Autodesk Fusion 360 part; units mm, degrees
(part 4 of 4)
sketch "Esboço11" plane through (0, 0, 2) normal (0, 0, 1) x (-1, 0, 0)
  circle A0 centre (10.25, -46.6) radius 1.5
  line L0 (8, -42.5) -> (8, -50.7)
  line L1 (8, -50.7) -> (-8, -50.7)
  line L2 (-8, -50.7) -> (-8, -42.5)
  line L3 (-8, -42.5) -> (8, -42.5)
  circle A1 centre (-10.25, -46.6) radius 1.5
  circle A2 centre (40.65, 50) radius 2.15
  arc A3 (-57.5607, 76.943) -> (-64.8173, 70.6939) centre (-60.2496, 72.7276) ccw
  line L4 (-57.5607, 76.943) -> (-49.4611, 71.7764)
  arc A4 (-47.15, 67.561) -> (-49.4611, 71.7764) centre (-52.15, 67.561) ccw
  line L5 (-47.15, 67.561) -> (-47.15, 42.4858)
  arc A5 (-47.4521, 41.7697) -> (-47.15, 42.4858) centre (-48.15, 42.4858) ccw
  line L6 (-47.4521, 41.7697) -> (-49.5538, 39.7214)
  arc A6 (-51.1653, 40.0309) -> (-49.5538, 39.7214) centre (-50.2517, 40.4376) ccw
  line L7 (-51.1653, 40.0309) -> (-64.8173, 70.6939)
  circle A7 centre (-40.65, 50) radius 2.15
  circle A8 centre (40.65, 60) radius 2.15
  line L8 (47.15, 42.4858) -> (47.15, 67.561)
  arc A9 (49.4611, 71.7764) -> (47.15, 67.561) centre (52.15, 67.561) ccw
  line L9 (49.4611, 71.7764) -> (57.5607, 76.943)
  arc A10 (64.8173, 70.6939) -> (57.5607, 76.943) centre (60.2496, 72.7276) ccw
  line L10 (64.8173, 70.6939) -> (51.1653, 40.0309)
  arc A11 (49.5538, 39.7214) -> (51.1653, 40.0309) centre (50.2517, 40.4376) ccw
  line L11 (49.5538, 39.7214) -> (47.4521, 41.7697)
  arc A12 (47.15, 42.4858) -> (47.4521, 41.7697) centre (48.15, 42.4858) ccw
  circle A13 centre (-40.65, 60) radius 2.15
  line L12 (-6.3787, 9) -> (6.3787, 9)
  arc A14 (6.7322, 8.1464) -> (6.3787, 9) centre (6.3787, 8.5) ccw
  line L13 (6.7322, 8.1464) -> (0.7071, 2.1213)
  arc A15 (-0.7071, 2.1213) -> (0.7071, 2.1213) centre (0, 2.8284) ccw
  line L14 (-0.7071, 2.1213) -> (-6.7322, 8.1464)
  arc A16 (-6.3787, 9) -> (-6.7322, 8.1464) centre (-6.3787, 8.5) ccw
  line L15 (-9, -6.3787) -> (-9, 6.3787)
  arc A17 (-8.1464, 6.7322) -> (-9, 6.3787) centre (-8.5, 6.3787) ccw
  line L16 (-8.1464, 6.7322) -> (-2.1213, 0.7071)
  arc A18 (-2.1213, -0.7071) -> (-2.1213, 0.7071) centre (-2.8284, 0) ccw
  line L17 (-2.1213, -0.7071) -> (-8.1464, -6.7322)
  arc A19 (-9, -6.3787) -> (-8.1464, -6.7322) centre (-8.5, -6.3787) ccw
  circle A20 centre (0, 87.5) radius 2.15
  line L18 (-16.4256, 75.2214) -> (0, 81.5)
  line L19 (0, 81.5) -> (15.6612, 75.3836)
  line L20 (41.7895, -17.0192) -> (61.9965, -63.6935)
  arc A21 (55.3948, -68.0303) -> (61.9965, -63.6935) centre (58.3475, -65.3318) ccw
  line L21 (55.3948, -68.0303) -> (23.5953, -33.2362)
  arc A22 (23.7067, -29.0729) -> (23.5953, -33.2362) centre (25.8097, -31.2123) ccw
  line L22 (23.7067, -29.0729) -> (36.9334, -16.0716)
  arc A23 (41.7895, -17.0192) -> (36.9334, -16.0716) centre (39.0364, -18.2111) ccw
  arc A24 (37.4337, 15.5639) -> (40.6601, 16.1647) centre (38.8376, 16.9884) ccw
  line L23 (37.4337, 15.5639) -> (14.6425, 38.0264)
  arc A25 (15.1963, 41.2612) -> (14.6425, 38.0264) centre (16.0464, 39.4508) ccw
  line L24 (15.1963, 41.2612) -> (28.3187, 47.4234)
  arc A26 (34.7856, 45.3775) -> (28.3187, 47.4234) centre (30.444, 42.8975) ccw
  arc A27 (34.7856, 45.3775) -> (44.4886, 35.8486) centre (56.4937, 57.7776) ccw
  arc A28 (46.6438, 29.4035) -> (44.4886, 35.8486) centre (42.0875, 31.4628) ccw
  line L25 (46.6438, 29.4035) -> (40.6601, 16.1647)
  arc A29 (9.266, 38.142) -> (7.6383, 38.7303) centre (7.8393, 36.7404) ccw
  line L26 (9.266, 38.142) -> (19.2664, 27.9622)
  arc A30 (17.8415, 24.5606) -> (19.2664, 27.9622) centre (17.8397, 26.5606) ccw
  line L27 (17.8415, 24.5606) -> (-17.871, 24.5283)
  arc A31 (-19.3052, 27.9241) -> (-17.871, 24.5283) centre (-17.8728, 26.5283) ccw
  line L28 (-19.3052, 27.9241) -> (-9.3455, 38.1438)
  arc A32 (-7.7103, 38.7376) -> (-9.3455, 38.1438) centre (-7.9132, 36.7479) ccw
  arc A33 (-7.7103, 38.7376) -> (7.6383, 38.7303) centre (0, 114.3455) ccw
  arc A34 (-40.9054, 16.7074) -> (-37.3489, 15.6517) centre (-38.8619, 17.0732) ccw
  line L29 (-40.9054, 16.7074) -> (-46.7322, 29.5993)
  arc A35 (-44.339, 36.0244) -> (-46.7322, 29.5993) centre (-42.0339, 31.5075) ccw
  arc A36 (-44.339, 36.0244) -> (-34.6129, 45.4956) centre (-56.2565, 57.9923) ccw
  arc A37 (-28.1234, 47.5076) -> (-34.6129, 45.4956) centre (-30.28, 42.9921) ccw
  line L30 (-28.1234, 47.5076) -> (-14.9942, 41.2515)
  arc A38 (-14.46, 38.0146) -> (-14.9942, 41.2515) centre (-15.8549, 39.4469) ccw
  line L31 (-14.46, 38.0146) -> (-37.3489, 15.6517)
  line L32 (19.3052, -27.9241) -> (9.3455, -38.1438)
  arc A39 (7.7103, -38.7376) -> (9.3455, -38.1438) centre (7.9132, -36.7479) ccw
  arc A40 (7.7103, -38.7376) -> (-7.6383, -38.7303) centre (0, -114.3455) ccw
  arc A41 (-9.266, -38.142) -> (-7.6383, -38.7303) centre (-7.8393, -36.7404) ccw
  line L33 (-9.266, -38.142) -> (-19.2664, -27.9622)
  arc A42 (-17.8415, -24.5606) -> (-19.2664, -27.9622) centre (-17.8397, -26.5606) ccw
  line L34 (-17.8415, -24.5606) -> (17.871, -24.5283)
  arc A43 (19.3052, -27.9241) -> (17.871, -24.5283) centre (17.8728, -26.5283) ccw
  arc A44 (-61.9967, -63.6938) -> (-55.4143, -68.0759) centre (-58.3695, -65.3802) ccw
  line L35 (-61.9967, -63.6938) -> (-41.8922, -17.2564)
  arc A45 (-36.246, -16.5772) -> (-41.8922, -17.2564) centre (-38.8636, -18.6251) ccw
  line L36 (-36.246, -16.5772) -> (-23.6374, -29.1331)
  arc A46 (-23.5625, -33.2372) -> (-23.6374, -29.1331) centre (-25.7596, -31.2246) ccw
  line L37 (-23.5625, -33.2372) -> (-55.4143, -68.0759)
  arc A47 (-38.7303, -7.6383) -> (-38.142, -9.266) centre (-36.7404, -7.8393) ccw
  arc A48 (-38.7303, -7.6383) -> (-38.7376, 7.7103) centre (-114.3455, 0) ccw
  arc A49 (-38.1438, 9.3455) -> (-38.7376, 7.7103) centre (-36.7479, 7.9132) ccw
  line L38 (-38.1438, 9.3455) -> (-27.9241, 19.3052)
  arc A50 (-24.5283, 17.871) -> (-27.9241, 19.3052) centre (-26.5283, 17.8728) ccw
  line L39 (-24.5283, 17.871) -> (-24.5606, -17.8415)
  arc A51 (-27.9622, -19.2664) -> (-24.5607, -17.8415) centre (-26.5606, -17.8397) ccw
  line L40 (-27.9622, -19.2664) -> (-38.142, -9.266)
  arc A52 (38.1376, -9.2791) -> (38.7256, -7.6527) centre (36.7356, -7.8528) ccw
  line L41 (38.1376, -9.2791) -> (27.9736, -19.2699)
  arc A53 (24.5716, -17.8424) -> (27.9736, -19.2699) centre (26.5716, -17.8436) ccw
  line L42 (24.5716, -17.8424) -> (24.5916, 17.8264)
  arc A54 (27.9955, 19.2498) -> (24.5916, 17.8264) centre (26.5916, 17.8253) ccw
  line L43 (27.9955, 19.2498) -> (38.1463, 9.2454)
  arc A55 (38.7321, 7.6192) -> (38.1463, 9.2454) centre (36.7424, 7.821) ccw
  arc A56 (38.7321, 7.6192) -> (38.7256, -7.6527) centre (114.3432, -0.0492) ccw
  line L44 (5, -97.464) -> (5, -58.6595)
  arc A57 (7, -56.6595) -> (5, -58.6595) centre (7, -58.6595) ccw
  line L45 (7, -56.6595) -> (10.473, -56.6595)
  arc A58 (14.3032, -58.4456) -> (10.473, -56.6595) centre (10.473, -61.6595) ccw
  line L46 (14.3032, -58.4456) -> (34.3305, -82.3132)
  arc A59 (35.4243, -86.3954) -> (34.3305, -82.3132) centre (30.5003, -85.5271) ccw
  line L47 (35.4243, -86.3954) -> (32.7648, -101.4781)
  arc A60 (26.9725, -105.5339) -> (32.7648, -101.4781) centre (27.8408, -100.6098) ccw
  line L48 (26.9725, -105.5339) -> (9.1318, -102.3881)
  arc A61 (5, -97.464) -> (9.1318, -102.3881) centre (10, -97.464) ccw
  arc A62 (8.1464, -6.7322) -> (9, -6.3787) centre (8.5, -6.3787) ccw
  line L49 (8.1464, -6.7322) -> (2.1213, -0.7071)
  arc A63 (2.1213, 0.7071) -> (2.1213, -0.7071) centre (2.8284, 0) ccw
  line L50 (2.1213, 0.7071) -> (8.1464, 6.7322)
  arc A64 (9, 6.3787) -> (8.1464, 6.7322) centre (8.5, 6.3787) ccw
  line L51 (9, 6.3787) -> (9, -6.3787)
  line L52 (6.3787, -9) -> (-6.3787, -9)
  arc A65 (-6.7322, -8.1464) -> (-6.3787, -9) centre (-6.3787, -8.5) ccw
  line L53 (-6.7322, -8.1464) -> (-0.7071, -2.1213)
  arc A66 (0.7071, -2.1213) -> (-0.7071, -2.1213) centre (0, -2.8284) ccw
  line L54 (0.7071, -2.1213) -> (6.7322, -8.1464)
  arc A67 (6.3787, -9) -> (6.7322, -8.1464) centre (6.3787, -8.5) ccw
  arc A68 (-10.473, -56.6595) -> (-14.3032, -58.4456) centre (-10.473, -61.6595) ccw
  line L55 (-10.473, -56.6595) -> (-7, -56.6595)
  arc A69 (-5, -58.6595) -> (-7, -56.6595) centre (-7, -58.6595) ccw
  line L56 (-5, -58.6595) -> (-5, -97.464)
  arc A70 (-9.1318, -102.3881) -> (-5, -97.464) centre (-10, -97.464) ccw
  line L57 (-9.1318, -102.3881) -> (-26.9725, -105.5339)
  arc A71 (-32.7648, -101.4781) -> (-26.9725, -105.5339) centre (-27.8408, -100.6098) ccw
  line L58 (-32.7648, -101.4781) -> (-35.4243, -86.3954)
  arc A72 (-34.3305, -82.3132) -> (-35.4243, -86.3954) centre (-30.5003, -85.5271) ccw
  line L59 (-34.3305, -82.3132) -> (-14.3032, -58.4456)
  circle A73 centre (72.5, -79.6021) radius 1.5
  circle A74 centre (72.5, -87.6021) radius 3
  circle A75 centre (-67, -87.4995) radius 1.5
  circle A76 centre (-74.9998, 79.5) radius 1.5
  circle A77 centre (67, 87.5) radius 1.5
  circle A78 centre (75, 87.5) radius 3
  circle A79 centre (75, 95.5) radius 1.5
  circle A80 centre (-83, 87.4998) radius 1.5
  circle A81 centre (-75, -87.5) radius 3
  circle A82 centre (80.5, -87.6021) radius 1.5
  circle A83 centre (64.5, -87.6021) radius 1.5
  circle A84 centre (-75.0005, -79.5) radius 1.5
  circle A85 centre (-74.9995, -95.5) radius 1.5
  circle A86 centre (-75, 87.5) radius 3
  circle A87 centre (75, 79.5) radius 1.5
  circle A88 centre (83, 87.5) radius 1.5
  circle A89 centre (-67, 87.5002) radius 1.5
  circle A90 centre (-75.0002, 95.5) radius 1.5
  circle A91 centre (-83, -87.5005) radius 1.5
  circle A92 centre (72.5, -95.6021) radius 1.5
  arc A93 (-89.8492, -89.6213) -> (-86.4551, -92.1669) centre (-86.8794, -89.1971) ccw
  arc A94 (-79.6669, -98.9551) -> (-86.4551, -92.1669) centre (-85.6066, -98.1066) ccw
  arc A95 (-79.6669, -98.9551) -> (-77.1213, -102.3492) centre (-76.6971, -99.3794) ccw
  arc A96 (-77.1213, -102.3492) -> (-73.7447, -102.4474) centre (-75, -87.5) ccw
  arc A97 (-46.7294, -108.889) -> (-73.7447, -102.4474) centre (-70.0264, -146.7235) ccw
  arc A98 (72.6915, -102.3213) -> (44.7852, -108.3244) centre (66.5604, -141.6847) ccw
  arc A99 (72.6915, -102.3213) -> (76.9019, -101.649) centre (72.5, -87.6021) ccw
  arc A100 (77.1213, -102.3492) -> (79.6669, -98.9551) centre (76.6971, -99.3794) ccw
  arc A101 (86.4551, -92.1669) -> (79.6669, -98.9551) centre (85.6066, -98.1066) ccw
  arc A102 (86.4551, -92.1669) -> (89.8492, -89.6213) centre (86.8794, -89.1971) ccw
  arc A103 (89.8492, -89.6213) -> (89.8247, -85.3818) centre (72.5, -87.6021) ccw
  arc A104 (89.8492, -85.3787) -> (86.4551, -82.8331) centre (86.8794, -85.8029) ccw
  arc A105 (79.7798, -75.4623) -> (86.4551, -82.8331) centre (85.6066, -76.8934) ccw
  arc A106 (79.7798, -75.4623) -> (78.5519, -72.265) centre (76.8663, -74.7468) ccw
  arc A107 (60.7593, -50.7677) -> (78.5519, -72.265) centre (106.6436, -30.9026) ccw
  line L60 (60.7593, -50.7677) -> (52.7268, -32.2145)
  arc A108 (51.9852, -22.4406) -> (52.7268, -32.2145) centre (66.4922, -26.2549) ccw
  arc A109 (51.9852, -22.4406) -> (52.0095, 23.4499) centre (-35.4576, 0.5509) ccw
  arc A110 (52.8518, 33.4268) -> (52.0095, 23.4499) centre (66.5205, 27.2489) ccw
  line L61 (52.8518, 33.4268) -> (60.9948, 51.443)
  arc A111 (78.5458, 72.2669) -> (60.9948, 51.443) centre (106.557, 30.8499) ccw
  arc A112 (78.5458, 72.2669) -> (79.7789, 75.4657) centre (76.8651, 74.7519) ccw
  arc A113 (86.4551, 82.8331) -> (79.7789, 75.4657) centre (85.6066, 76.8934) ccw
  arc A114 (86.4551, 82.8331) -> (89.8492, 85.3787) centre (86.8794, 85.8029) ccw
  arc A115 (89.8492, 85.3787) -> (89.8492, 89.6213) centre (75, 87.5) ccw
  arc A116 (89.8492, 89.6213) -> (86.4551, 92.1669) centre (86.8794, 89.1971) ccw
  arc A117 (79.6669, 98.9551) -> (86.4551, 92.1669) centre (85.6066, 98.1066) ccw
  arc A118 (79.6669, 98.9551) -> (77.1213, 102.3492) centre (76.6971, 99.3794) ccw
  arc A119 (77.1213, 102.3492) -> (72.8787, 102.3492) centre (75, 87.5) ccw
  arc A120 (72.8787, 102.3492) -> (70.3331, 98.9551) centre (73.3029, 99.3794) ccw
  arc A121 (62.5456, 92.3982) -> (70.3331, 98.9551) centre (64.3934, 98.1066) ccw
  arc A122 (62.5456, 92.3982) -> (59.6541, 91.8087) centre (61.6216, 89.544) ccw
  arc A123 (44.4663, 82.7551) -> (59.6541, 91.8087) centre (26.8616, 129.5533) ccw
  line L62 (35.9657, 79.8952) -> (2.1827, 93.0889)
  arc A124 (2.1827, 93.0889) -> (-2.1423, 93.1045) centre (0, 87.5) ccw
  line L63 (-2.1423, 93.1045) -> (-36.9275, 79.8081)
  arc A125 (-59.6538, 91.7779) -> (-44.9685, 82.7086) centre (-26.4329, 129.146) ccw
  arc A126 (-59.6538, 91.7779) -> (-62.5625, 92.3928) centre (-61.6471, 89.5359) ccw
  arc A127 (-70.3331, 98.9551) -> (-62.5625, 92.3928) centre (-64.3934, 98.1066) ccw
  arc A128 (-70.3331, 98.9551) -> (-72.8787, 102.3492) centre (-73.3029, 99.3794) ccw
  arc A129 (-72.8787, 102.3492) -> (-77.1213, 102.3492) centre (-75, 87.5) ccw
  arc A130 (-77.1213, 102.3492) -> (-79.6669, 98.9551) centre (-76.6971, 99.3794) ccw
  arc A131 (-86.4551, 92.1669) -> (-79.6669, 98.9551) centre (-85.6066, 98.1066) ccw
  arc A132 (-86.4551, 92.1669) -> (-89.8492, 89.6213) centre (-86.8794, 89.1971) ccw
  arc A133 (-89.8492, 89.6213) -> (-89.8492, 85.3787) centre (-75, 87.5) ccw
  arc A134 (-89.8492, 85.3787) -> (-86.4551, 82.8331) centre (-86.8794, 85.8029) ccw
  arc A135 (-79.7789, 75.4657) -> (-86.4551, 82.8331) centre (-85.6066, 76.8934) ccw
  arc A136 (-79.7789, 75.4657) -> (-78.5458, 72.2669) centre (-76.8651, 74.7519) ccw
  arc A137 (-60.9948, 51.443) -> (-78.5458, 72.2669) centre (-106.557, 30.8499) ccw
  line L64 (-60.9948, 51.443) -> (-52.8518, 33.4268)
  arc A138 (-52.0095, 23.4499) -> (-52.8518, 33.4268) centre (-66.5205, 27.2489) ccw
  arc A139 (-52.0095, 23.4499) -> (-51.9852, -22.4406) centre (35.4576, 0.5509) ccw
  arc A140 (-52.7268, -32.2145) -> (-51.9852, -22.4406) centre (-66.4922, -26.2549) ccw
  line L65 (-52.7268, -32.2145) -> (-60.7593, -50.7677)
  arc A141 (-78.5519, -72.265) -> (-60.7593, -50.7677) centre (-106.6436, -30.9026) ccw
  arc A142 (-78.5519, -72.265) -> (-79.7798, -75.4623) centre (-76.8663, -74.7468) ccw
  arc A143 (-86.4551, -82.8331) -> (-79.7798, -75.4623) centre (-85.6066, -76.8934) ccw
  arc A144 (-86.4551, -82.8331) -> (-89.8492, -85.3787) centre (-86.8794, -85.8029) ccw
  arc A145 (-89.8492, -85.3787) -> (-89.8492, -89.6213) centre (-75, -87.5) ccw
  circle A146 centre (50, 0) radius 2.15
  circle A147 centre (-50, 0) radius 2.15
  circle A148 centre (0, -87.5) radius 2.15
  circle A149 centre (42, -73) radius 2.15
  circle A150 centre (-42, -73) radius 2.15
  line L66 (0, 0) -> (0, -160) construction
  arc A151 (26.2105, 50.915) -> (27.5676, 55.0697) centre (24.9353, 53.6305) ccw
  line L67 (26.2105, 50.915) -> (10.6059, 43.5872)
  arc A152 (9.3307, 43.3027) -> (10.6059, 43.5872) centre (9.3307, 46.3027) ccw
  line L68 (9.3307, 43.3027) -> (-9.3218, 43.3027)
  arc A153 (-10.6123, 43.5944) -> (-9.3218, 43.3027) centre (-9.3218, 46.3027) ccw
  line L69 (-10.6123, 43.5944) -> (-26.8632, 51.3381)
  arc A154 (-28.1945, 55.5044) -> (-26.8632, 51.3381) centre (-25.5727, 54.0463) ccw
  line L70 (-28.1945, 55.5044) -> (-17.9762, 73.8773)
  arc A155 (-16.4256, 75.2214) -> (-17.9762, 73.8773) centre (-15.3544, 72.4192) ccw
  arc A156 (17.2021, 74.0283) -> (15.6612, 75.3836) centre (14.5698, 72.5892) ccw
  line L71 (17.2021, 74.0283) -> (27.5676, 55.0697)
  arc A157 (-46.7294, -108.889) -> (-25.7561, -114.8285) centre (-25.7561, -74.8285) ccw
  line L72 (-25.7561, -114.8285) -> (22.9214, -114.8285)
  arc A158 (22.9214, -114.8285) -> (44.7852, -108.3244) centre (22.9214, -74.8285) ccw
  circle A159 centre (10, 10) radius 3
  circle A160 centre (-10, -10) radius 3
  circle A161 centre (10, -10) radius 3
  circle A162 centre (-10, 10) radius 3
  arc A163 (35.9657, 79.8952) -> (44.4663, 82.7551) centre (-0.31, 201.7835) ccw
  arc A164 (-44.9685, 82.7086) -> (-36.9275, 79.8081) centre (2.2046, 200.8918) ccw
  point P0 (-72.5, -87.5)
  point P1 (72.5, -87.5)
  point P2 (72.5, 87.5)
  point P3 (-72.5, 87.5)
  point P4 (-72.5, -87.5)
  point P5 (72.5, -87.5)
  point P6 (72.5, 87.5)
  point P7 (-72.5, 87.5)
  point P8 (-72.5, -87.5)
  point P9 (72.5, -87.5)
  point P10 (72.5, 87.5)
  point P11 (-72.5, 87.5)
  point P12 (72.5, -87.5)
  point P13 (75, -87.7706)
  point P14 (75, -87.7706)
  point P15 (75, -87.7706)
  point P16 (75, -87.7706)
  point P17 (75, -87.5)
  dimension "d158" = 4.3
  dimension "d159" = 4.3
  dimension "d160" = 73
  dimension "d161" = 42
  constraint coincident L66.start origin
  constraint perpendicular L52 L66
  constraint symmetric A149 A150 L66
  measures "d158" diameter of A149
  measures "d159" diameter of A150
  measures "d160" vertical distance of L66.start A149.centre
  measures "d161" distance of A149.centre L66
extrude "Extrusão10" cut sketch "Esboço11" against normal through all contours A149 | A150
sketch "Esboço12" plane through (0, 0, 2) normal (0, 0, 1) x (-1, 0, 0)
  circle A0 centre (0, -87.5) radius 2.15
  circle A1 centre (-50, 0) radius 2.15
  circle A2 centre (50, 0) radius 2.15
  arc A3 (-89.8492, -89.6213) -> (-86.4551, -92.1669) centre (-86.8794, -89.1971) ccw
  arc A4 (-79.6669, -98.9551) -> (-86.4551, -92.1669) centre (-85.6066, -98.1066) ccw
  arc A5 (-79.6669, -98.9551) -> (-77.1213, -102.3492) centre (-76.6971, -99.3794) ccw
  arc A6 (-77.1213, -102.3492) -> (-73.7447, -102.4474) centre (-75, -87.5) ccw
  arc A7 (-46.7294, -108.889) -> (-73.7447, -102.4474) centre (-70.0264, -146.7235) ccw
  arc A8 (-46.7294, -108.889) -> (-25.7561, -114.8285) centre (-25.7561, -74.8285) ccw
  line L0 (-25.7561, -114.8285) -> (22.9214, -114.8285)
  arc A9 (22.9214, -114.8285) -> (44.7852, -108.3244) centre (22.9214, -74.8285) ccw
  arc A10 (72.6915, -102.3213) -> (44.7852, -108.3244) centre (66.5604, -141.6847) ccw
  arc A11 (72.6915, -102.3213) -> (77.1213, -102.3492) centre (75, -87.5) ccw
  arc A12 (77.1213, -102.3492) -> (79.6669, -98.9551) centre (76.6971, -99.3794) ccw
  arc A13 (86.4551, -92.1669) -> (79.6669, -98.9551) centre (85.6066, -98.1066) ccw
  arc A14 (86.4551, -92.1669) -> (89.8492, -89.6213) centre (86.8794, -89.1971) ccw
  arc A15 (89.8492, -89.6213) -> (89.8492, -85.3787) centre (75, -87.5) ccw
  arc A16 (89.8492, -85.3787) -> (86.4551, -82.8331) centre (86.8794, -85.8029) ccw
  arc A17 (79.7798, -75.4623) -> (86.4551, -82.8331) centre (85.6066, -76.8934) ccw
  arc A18 (79.7798, -75.4623) -> (78.5519, -72.265) centre (76.8663, -74.7468) ccw
  arc A19 (60.7593, -50.7677) -> (78.5519, -72.265) centre (106.6436, -30.9026) ccw
  line L1 (60.7593, -50.7677) -> (52.7268, -32.2145)
  arc A20 (51.9852, -22.4406) -> (52.7268, -32.2145) centre (66.4922, -26.2549) ccw
  arc A21 (51.9852, -22.4406) -> (52.0095, 23.4499) centre (-35.4576, 0.5509) ccw
  arc A22 (52.8518, 33.4268) -> (52.0095, 23.4499) centre (66.5205, 27.2489) ccw
  line L2 (52.8518, 33.4268) -> (60.9948, 51.443)
  arc A23 (78.5458, 72.2669) -> (60.9948, 51.443) centre (106.557, 30.8499) ccw
  arc A24 (78.5458, 72.2669) -> (79.7789, 75.4657) centre (76.8651, 74.7519) ccw
  arc A25 (86.4551, 82.8331) -> (79.7789, 75.4657) centre (85.6066, 76.8934) ccw
  arc A26 (86.4551, 82.8331) -> (89.8492, 85.3787) centre (86.8794, 85.8029) ccw
  arc A27 (89.8492, 85.3787) -> (89.8492, 89.6213) centre (75, 87.5) ccw
  arc A28 (89.8492, 89.6213) -> (86.4551, 92.1669) centre (86.8794, 89.1971) ccw
  arc A29 (79.6669, 98.9551) -> (86.4551, 92.1669) centre (85.6066, 98.1066) ccw
  arc A30 (79.6669, 98.9551) -> (77.1213, 102.3492) centre (76.6971, 99.3794) ccw
  arc A31 (77.1213, 102.3492) -> (72.8787, 102.3492) centre (75, 87.5) ccw
  arc A32 (72.8787, 102.3492) -> (70.3331, 98.9551) centre (73.3029, 99.3794) ccw
  arc A33 (62.5456, 92.3982) -> (70.3331, 98.9551) centre (64.3934, 98.1066) ccw
  arc A34 (62.5456, 92.3982) -> (59.6541, 91.8087) centre (61.6216, 89.544) ccw
  arc A35 (44.4663, 82.7551) -> (59.6541, 91.8087) centre (26.8616, 129.5533) ccw
  line L3 (35.9657, 79.8952) -> (2.1827, 93.0889)
  arc A36 (2.1827, 93.0889) -> (-2.1423, 93.1045) centre (0, 87.5) ccw
  line L4 (-2.1423, 93.1045) -> (-36.9275, 79.8081)
  arc A37 (-59.6538, 91.7779) -> (-44.9685, 82.7086) centre (-26.4329, 129.146) ccw
  arc A38 (-59.6538, 91.7779) -> (-62.5625, 92.3928) centre (-61.6471, 89.5359) ccw
  arc A39 (-70.3331, 98.9551) -> (-62.5625, 92.3928) centre (-64.3934, 98.1066) ccw
  arc A40 (-70.3331, 98.9551) -> (-72.8787, 102.3492) centre (-73.3029, 99.3794) ccw
  arc A41 (-72.8787, 102.3492) -> (-77.1213, 102.3492) centre (-75, 87.5) ccw
  arc A42 (-77.1213, 102.3492) -> (-79.6669, 98.9551) centre (-76.6971, 99.3794) ccw
  arc A43 (-86.4551, 92.1669) -> (-79.6669, 98.9551) centre (-85.6066, 98.1066) ccw
  arc A44 (-86.4551, 92.1669) -> (-89.8492, 89.6213) centre (-86.8794, 89.1971) ccw
  arc A45 (-89.8492, 89.6213) -> (-89.8492, 85.3787) centre (-75, 87.5) ccw
  arc A46 (-89.8492, 85.3787) -> (-86.4551, 82.8331) centre (-86.8794, 85.8029) ccw
  arc A47 (-79.7789, 75.4657) -> (-86.4551, 82.8331) centre (-85.6066, 76.8934) ccw
  arc A48 (-79.7789, 75.4657) -> (-78.5458, 72.2669) centre (-76.8651, 74.7519) ccw
  arc A49 (-60.9948, 51.443) -> (-78.5458, 72.2669) centre (-106.557, 30.8499) ccw
  line L5 (-60.9948, 51.443) -> (-52.8518, 33.4268)
  arc A50 (-52.0095, 23.4499) -> (-52.8518, 33.4268) centre (-66.5205, 27.2489) ccw
  arc A51 (-52.0095, 23.4499) -> (-51.9852, -22.4406) centre (35.4576, 0.5509) ccw
  arc A52 (-52.7268, -32.2145) -> (-51.9852, -22.4406) centre (-66.4922, -26.2549) ccw
  line L6 (-52.7268, -32.2145) -> (-60.7593, -50.7677)
  arc A53 (-78.5519, -72.265) -> (-60.7593, -50.7677) centre (-106.6436, -30.9026) ccw
  arc A54 (-78.5519, -72.265) -> (-79.7798, -75.4623) centre (-76.8663, -74.7468) ccw
  arc A55 (-86.4551, -82.8331) -> (-79.7798, -75.4623) centre (-85.6066, -76.8934) ccw
  arc A56 (-86.4551, -82.8331) -> (-89.8492, -85.3787) centre (-86.8794, -85.8029) ccw
  arc A57 (-89.8492, -85.3787) -> (-89.8492, -89.6213) centre (-75, -87.5) ccw
  circle A58 centre (72.5, -95.6021) radius 1.5
  circle A59 centre (-83, -87.5005) radius 1.5
  circle A60 centre (-75.0002, 95.5) radius 1.5
  circle A61 centre (-67, 87.5002) radius 1.5
  circle A62 centre (83, 87.5) radius 1.5
  circle A63 centre (75, 79.5) radius 1.5
  circle A64 centre (-75, 87.5) radius 3
  circle A65 centre (-74.9995, -95.5) radius 1.5
  circle A66 centre (-75.0005, -79.5) radius 1.5
  circle A67 centre (64.5, -87.6021) radius 1.5
  circle A68 centre (80.5, -87.6021) radius 1.5
  circle A69 centre (-75, -87.5) radius 3
  circle A70 centre (-83, 87.4998) radius 1.5
  circle A71 centre (75, 95.5) radius 1.5
  circle A72 centre (75, 87.5) radius 3
  circle A73 centre (67, 87.5) radius 1.5
  circle A74 centre (-74.9998, 79.5) radius 1.5
  circle A75 centre (-67, -87.4995) radius 1.5
  circle A76 centre (75, -87.5) radius 3
  circle A77 centre (72.5, -79.6021) radius 1.5
  line L7 (-10.473, -56.6595) -> (-7, -56.6595)
  arc A78 (-5, -58.6595) -> (-7, -56.6595) centre (-7, -58.6595) ccw
  line L8 (-5, -58.6595) -> (-5, -97.464)
  arc A79 (-9.1318, -102.3881) -> (-5, -97.464) centre (-10, -97.464) ccw
  line L9 (-9.1318, -102.3881) -> (-26.9725, -105.5339)
  arc A80 (-32.7648, -101.4781) -> (-26.9725, -105.5339) centre (-27.8408, -100.6098) ccw
  line L10 (-32.7648, -101.4781) -> (-35.4243, -86.3954)
  arc A81 (-34.3305, -82.3132) -> (-35.4243, -86.3954) centre (-30.5003, -85.5271) ccw
  line L11 (-34.3305, -82.3132) -> (-14.3032, -58.4456)
  arc A82 (-10.473, -56.6595) -> (-14.3032, -58.4456) centre (-10.473, -61.6595) ccw
  arc A83 (7, -56.6595) -> (5, -58.6595) centre (7, -58.6595) ccw
  line L12 (7, -56.6595) -> (10.473, -56.6595)
  arc A84 (14.3032, -58.4456) -> (10.473, -56.6595) centre (10.473, -61.6595) ccw
  line L13 (14.3032, -58.4456) -> (34.3305, -82.3132)
  arc A85 (35.4243, -86.3954) -> (34.3305, -82.3132) centre (30.5003, -85.5271) ccw
  line L14 (35.4243, -86.3954) -> (32.7648, -101.4781)
  arc A86 (26.9725, -105.5339) -> (32.7648, -101.4781) centre (27.8408, -100.6098) ccw
  line L15 (26.9725, -105.5339) -> (9.1318, -102.3881)
  arc A87 (5, -97.464) -> (9.1318, -102.3881) centre (10, -97.464) ccw
  line L16 (5, -97.464) -> (5, -58.6595)
  line L17 (-40.9054, 16.7074) -> (-46.7322, 29.5993)
  arc A88 (-44.339, 36.0244) -> (-46.7322, 29.5993) centre (-42.0339, 31.5075) ccw
  arc A89 (-44.339, 36.0244) -> (-34.6129, 45.4956) centre (-56.2565, 57.9923) ccw
  arc A90 (-28.1234, 47.5076) -> (-34.6129, 45.4956) centre (-30.28, 42.9921) ccw
  line L18 (-28.1234, 47.5076) -> (-14.9942, 41.2515)
  arc A91 (-14.46, 38.0146) -> (-14.9942, 41.2515) centre (-15.8549, 39.4469) ccw
  line L19 (-14.46, 38.0146) -> (-37.3489, 15.6517)
  arc A92 (-40.9054, 16.7074) -> (-37.3489, 15.6517) centre (-38.8619, 17.0732) ccw
  line L20 (37.4337, 15.5639) -> (14.6425, 38.0264)
  arc A93 (15.1963, 41.2612) -> (14.6425, 38.0264) centre (16.0464, 39.4508) ccw
  line L21 (15.1963, 41.2612) -> (28.3187, 47.4234)
  arc A94 (34.7856, 45.3775) -> (28.3187, 47.4234) centre (30.444, 42.8975) ccw
  arc A95 (34.7856, 45.3775) -> (44.4886, 35.8486) centre (56.4937, 57.7776) ccw
  arc A96 (46.6438, 29.4035) -> (44.4886, 35.8486) centre (42.0875, 31.4628) ccw
  line L22 (46.6438, 29.4035) -> (40.6601, 16.1647)
  arc A97 (37.4337, 15.5639) -> (40.6601, 16.1647) centre (38.8376, 16.9884) ccw
  line L23 (38.1376, -9.2791) -> (27.9736, -19.2699)
  arc A98 (24.5716, -17.8424) -> (27.9736, -19.2699) centre (26.5716, -17.8436) ccw
  line L24 (24.5716, -17.8424) -> (24.5916, 17.8264)
  arc A99 (27.9955, 19.2498) -> (24.5916, 17.8264) centre (26.5916, 17.8253) ccw
  line L25 (27.9955, 19.2498) -> (38.1463, 9.2454)
  arc A100 (38.7321, 7.6192) -> (38.1463, 9.2454) centre (36.7424, 7.821) ccw
  arc A101 (38.7321, 7.6192) -> (38.7256, -7.6527) centre (114.3432, -0.0492) ccw
  arc A102 (38.1376, -9.2791) -> (38.7256, -7.6527) centre (36.7356, -7.8528) ccw
  line L26 (9.266, 38.142) -> (19.2664, 27.9622)
  arc A103 (17.8415, 24.5606) -> (19.2664, 27.9622) centre (17.8397, 26.5606) ccw
  line L27 (17.8415, 24.5606) -> (-17.871, 24.5283)
  arc A104 (-19.3052, 27.9241) -> (-17.871, 24.5283) centre (-17.8728, 26.5283) ccw
  line L28 (-19.3052, 27.9241) -> (-9.3455, 38.1438)
  arc A105 (-7.7103, 38.7376) -> (-9.3455, 38.1438) centre (-7.9132, 36.7479) ccw
  arc A106 (-7.7103, 38.7376) -> (7.6383, 38.7303) centre (0, 114.3455) ccw
  arc A107 (9.266, 38.142) -> (7.6383, 38.7303) centre (7.8393, 36.7404) ccw
  arc A108 (-38.7303, -7.6383) -> (-38.7376, 7.7103) centre (-114.3455, 0) ccw
  arc A109 (-38.1438, 9.3455) -> (-38.7376, 7.7103) centre (-36.7479, 7.9132) ccw
  line L29 (-38.1438, 9.3455) -> (-27.9241, 19.3052)
  arc A110 (-24.5283, 17.871) -> (-27.9241, 19.3052) centre (-26.5283, 17.8728) ccw
  line L30 (-24.5283, 17.871) -> (-24.5606, -17.8415)
  arc A111 (-27.9622, -19.2664) -> (-24.5607, -17.8415) centre (-26.5606, -17.8397) ccw
  line L31 (-27.9622, -19.2664) -> (-38.142, -9.266)
  arc A112 (-38.7303, -7.6383) -> (-38.142, -9.266) centre (-36.7404, -7.8393) ccw
  line L32 (-61.9967, -63.6938) -> (-41.8922, -17.2564)
  arc A113 (-36.246, -16.5772) -> (-41.8922, -17.2564) centre (-38.8636, -18.6251) ccw
  line L33 (-36.246, -16.5772) -> (-23.6374, -29.1331)
  arc A114 (-23.5625, -33.2372) -> (-23.6374, -29.1331) centre (-25.7596, -31.2246) ccw
  line L34 (-23.5625, -33.2372) -> (-55.4143, -68.0759)
  arc A115 (-61.9967, -63.6938) -> (-55.4143, -68.0759) centre (-58.3695, -65.3802) ccw
  arc A116 (7.7103, -38.7376) -> (9.3455, -38.1438) centre (7.9132, -36.7479) ccw
  arc A117 (7.7103, -38.7376) -> (-7.6383, -38.7303) centre (0, -114.3455) ccw
  arc A118 (-9.266, -38.142) -> (-7.6383, -38.7303) centre (-7.8393, -36.7404) ccw
  line L35 (-9.266, -38.142) -> (-19.2664, -27.9622)
  arc A119 (-17.8415, -24.5606) -> (-19.2664, -27.9622) centre (-17.8397, -26.5606) ccw
  line L36 (-17.8415, -24.5606) -> (17.871, -24.5283)
  arc A120 (19.3052, -27.9241) -> (17.871, -24.5283) centre (17.8728, -26.5283) ccw
  line L37 (19.3052, -27.9241) -> (9.3455, -38.1438)
  line L38 (23.7067, -29.0729) -> (36.9334, -16.0716)
  arc A121 (41.7895, -17.0192) -> (36.9334, -16.0716) centre (39.0364, -18.2111) ccw
  line L39 (41.7895, -17.0192) -> (61.9965, -63.6935)
  arc A122 (55.3948, -68.0303) -> (61.9965, -63.6935) centre (58.3475, -65.3318) ccw
  line L40 (55.3948, -68.0303) -> (23.5953, -33.2362)
  arc A123 (23.7067, -29.0729) -> (23.5953, -33.2362) centre (25.8097, -31.2123) ccw
  line L41 (-9, -6.3787) -> (-9, 6.3787)
  arc A124 (-8.1464, 6.7322) -> (-9, 6.3787) centre (-8.5, 6.3787) ccw
  line L42 (-8.1464, 6.7322) -> (-2.1213, 0.7071)
  arc A125 (-2.1213, -0.7071) -> (-2.1213, 0.7071) centre (-2.8284, 0) ccw
  line L43 (-2.1213, -0.7071) -> (-8.1464, -6.7322)
  arc A126 (-9, -6.3787) -> (-8.1464, -6.7322) centre (-8.5, -6.3787) ccw
  line L44 (-6.3787, 9) -> (6.3787, 9)
  arc A127 (6.7322, 8.1464) -> (6.3787, 9) centre (6.3787, 8.5) ccw
  line L45 (6.7322, 8.1464) -> (0.7071, 2.1213)
  arc A128 (-0.7071, 2.1213) -> (0.7071, 2.1213) centre (0, 2.8284) ccw
  line L46 (-0.7071, 2.1213) -> (-6.7322, 8.1464)
  arc A129 (-6.3787, 9) -> (-6.7322, 8.1464) centre (-6.3787, 8.5) ccw
  arc A130 (8.1464, -6.7322) -> (9, -6.3787) centre (8.5, -6.3787) ccw
  line L47 (8.1464, -6.7322) -> (2.1213, -0.7071)
  arc A131 (2.1213, 0.7071) -> (2.1213, -0.7071) centre (2.8284, 0) ccw
  line L48 (2.1213, 0.7071) -> (8.1464, 6.7322)
  arc A132 (9, 6.3787) -> (8.1464, 6.7322) centre (8.5, 6.3787) ccw
  line L49 (9, 6.3787) -> (9, -6.3787)
  line L50 (6.3787, -9) -> (-6.3787, -9)
  arc A133 (-6.7322, -8.1464) -> (-6.3787, -9) centre (-6.3787, -8.5) ccw
  line L51 (-6.7322, -8.1464) -> (-0.7071, -2.1213)
  arc A134 (0.7071, -2.1213) -> (-0.7071, -2.1213) centre (0, -2.8284) ccw
  line L52 (0.7071, -2.1213) -> (6.7322, -8.1464)
  arc A135 (6.3787, -9) -> (6.7322, -8.1464) centre (6.3787, -8.5) ccw
  circle A136 centre (0, 87.5) radius 2.15
  line L53 (0, 81.5) -> (15.6612, 75.3836)
  arc A137 (17.2021, 74.0283) -> (15.6612, 75.3836) centre (14.5698, 72.5892) ccw
  line L54 (17.2021, 74.0283) -> (27.5676, 55.0697)
  arc A138 (26.2105, 50.915) -> (27.5676, 55.0697) centre (24.9353, 53.6305) ccw
  line L55 (26.2105, 50.915) -> (10.6059, 43.5872)
  arc A139 (9.3307, 43.3027) -> (10.6059, 43.5872) centre (9.3307, 46.3027) ccw
  line L56 (9.3307, 43.3027) -> (-9.3218, 43.3027)
  arc A140 (-10.6123, 43.5944) -> (-9.3218, 43.3027) centre (-9.3218, 46.3027) ccw
  line L57 (-10.6123, 43.5944) -> (-26.8632, 51.3381)
  arc A141 (-28.1945, 55.5044) -> (-26.8632, 51.3381) centre (-25.5727, 54.0463) ccw
  line L58 (-28.1945, 55.5044) -> (-17.9762, 73.8773)
  arc A142 (-16.4256, 75.2214) -> (-17.9762, 73.8773) centre (-15.3544, 72.4192) ccw
  line L59 (-16.4256, 75.2214) -> (0, 81.5)
  circle A143 centre (-40.65, 60) radius 2.15
  line L60 (47.15, 42.4858) -> (47.15, 67.561)
  arc A144 (49.4611, 71.7764) -> (47.15, 67.561) centre (52.15, 67.561) ccw
  line L61 (49.4611, 71.7764) -> (57.5607, 76.943)
  arc A145 (64.8173, 70.6939) -> (57.5607, 76.943) centre (60.2496, 72.7276) ccw
  line L62 (64.8173, 70.6939) -> (51.1653, 40.0309)
  arc A146 (49.5538, 39.7214) -> (51.1653, 40.0309) centre (50.2517, 40.4376) ccw
  line L63 (49.5538, 39.7214) -> (47.4521, 41.7697)
  arc A147 (47.15, 42.4858) -> (47.4521, 41.7697) centre (48.15, 42.4858) ccw
  circle A148 centre (40.65, 60) radius 2.15
  circle A149 centre (-40.65, 50) radius 2.15
  arc A150 (-57.5607, 76.943) -> (-64.8173, 70.6939) centre (-60.2496, 72.7276) ccw
  line L64 (-57.5607, 76.943) -> (-49.4611, 71.7764)
  arc A151 (-47.15, 67.561) -> (-49.4611, 71.7764) centre (-52.15, 67.561) ccw
  line L65 (-47.15, 67.561) -> (-47.15, 42.4858)
  arc A152 (-47.4521, 41.7697) -> (-47.15, 42.4858) centre (-48.15, 42.4858) ccw
  line L66 (-47.4521, 41.7697) -> (-49.5538, 39.7214)
  arc A153 (-51.1653, 40.0309) -> (-49.5538, 39.7214) centre (-50.2517, 40.4376) ccw
  line L67 (-51.1653, 40.0309) -> (-64.8173, 70.6939)
  circle A154 centre (40.65, 50) radius 2.15
  circle A155 centre (-10.25, -46.6) radius 1.5
  line L68 (8, -42.5) -> (8, -50.7)
  line L69 (8, -50.7) -> (-8, -50.7)
  line L70 (-8, -50.7) -> (-8, -42.5)
  line L71 (-8, -42.5) -> (8, -42.5)
  circle A156 centre (10.25, -46.6) radius 1.5
  circle A157 centre (-42, -73) radius 2.15
  circle A158 centre (42, -73) radius 2.15
  circle A159 centre (-10, 10) radius 3
  circle A160 centre (10, -10) radius 3
  circle A161 centre (-10, -10) radius 3
  circle A162 centre (10, 10) radius 3
  arc A163 (35.9657, 79.8952) -> (44.4663, 82.7551) centre (-0.31, 201.7835) ccw
  arc A164 (-44.9685, 82.7086) -> (-36.9275, 79.8081) centre (2.2046, 200.8918) ccw
  point P0 (-72.5, 87.3979)
  point P1 (72.5, 87.3979)
  point P2 (72.5, -87.6021)
  point P3 (-72.5, 87.3979)
  point P4 (-72.5, -87.6021)
  point P5 (72.5, 87.3979)
  point P6 (72.5, -87.6021)
  point P7 (-72.5, 87.3979)
  point P8 (-72.5, -87.6021)
  point P9 (72.5, 87.3979)
  point P10 (72.5, -87.6021)
  point P11 (72.5, -87.6021)
  point P12 (72.5, -87.6021)
  point P13 (72.5, -87.6021)
  point P14 (72.5, -87.6021)
  point P15 (72.5, -87.6021)
  point P16 (72.5, -87.6021)
  dimension "d179" = 87.5
  dimension "d180" = 147.5
  dimension "d181" = 72.5
  dimension "d182" = 75
  dimension "d183" = 87.5
  dimension "d184" = 87.5
  dimension "d185" = 87.5
  measures "d179" vertical distance of origin A41.centre
  measures "d180" horizontal distance of A41.centre P9
  measures "d181" horizontal distance of origin P7
  measures "d182" horizontal distance of origin A6.centre
  measures "d183" distance of origin A0.centre
  measures "d184" distance of origin A36.centre
  measures "d185" vertical distance of origin A6.centre
fillet "Arredondamento5" radius 25 2 edges at (36.9275, -79.8081, 0) (-35.9657, -79.8952, 0)
equation "d173 = ( 175 / 2 ) * 1 mm"
